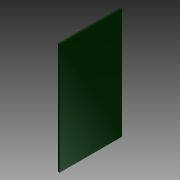
# Autodesk Inventor part: PowerPCB01
Saved by Autodesk Inventor 2015 (Build 190159000, 159)
## iProperties
Created: 2015-02-22
Part Number: PowerPCB01
Material: PCB
Document SubType Name: Modeling
Designer: spichelh
Density: 1 g/cm^3
Appearance: Smooth - White(1)
Author: spichelh
Autodesk Inventor part; units mm, degrees
ref_plane "YZ Plane" through (0, 0, 0) normal (1, 0, 0) x (0, 1, 0)
ref_plane "XZ Plane" through (0, 0, 0) normal (0, 1, 0) x (-1, 0, 0)
ref_plane "XY Plane" through (0, 0, 0) normal (0, 0, 1) x (1, 0, 0)
sketch "Sketch1" plane through (0, 0, 0) normal (1, 0, 0) x (0, 1, 0)
  line L0 (-50.8, 28.575) -> (50.8, 28.575)
  line L1 (50.8, 28.575) -> (50.8, -28.575)
  line L2 (50.8, -28.575) -> (-50.8, -28.575)
  line L3 (-50.8, -28.575) -> (-50.8, 28.575)
  line L4 (-50.8, 0) -> (50.8, 0) construction
  line L5 (0, 28.575) -> (0, -28.575) construction
  point P0 (0, 0)
  dimension "d0" = 101.6
  dimension "d2" = 57.15
  constraints: 12 end point, 6 midpoint, 2 parallel, 1 horizontal, 1 perpendicular
  measures "d0" distance of L0.start L0.end
  measures "d2" distance of L2.end L0.start
extrude "Extrusion1" add sketch "Sketch1" along normal blind 1.64
body "Solid1"
